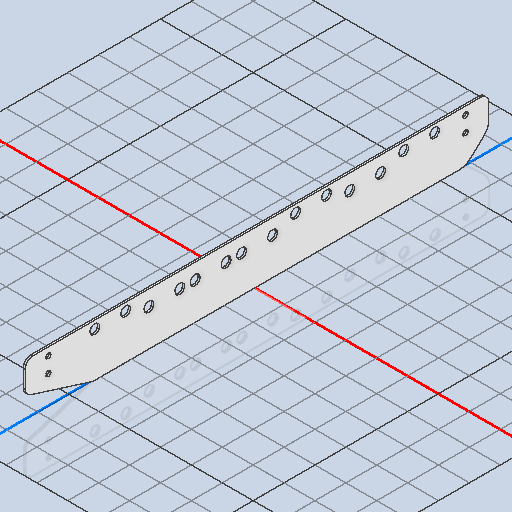
# Autodesk Inventor part: Skirt
Saved by Autodesk Inventor 2026 (Build 300175000, 175)
## iProperties
Created: 2025-04-07
Part Number: Skirt
Material: Acetal Resin, White
Document SubType Name: Modeling
Designer: avere
Density: 1.425 g/cm^3
Appearance: Smooth - White
Author: avere
Autodesk Inventor part; units mm, degrees
ref_plane "YZ Plane" through (0, 0, 0) normal (1, 0, 0) x (0, 1, 0)
ref_plane "XZ Plane" through (0, 0, 0) normal (0, 1, 0) x (-1, 0, 0)
ref_plane "XY Plane" through (0, 0, 0) normal (0, 0, 1) x (1, 0, 0)
sketch "Sketch1" plane through (0, 0, 0) normal (1, 0, 0) x (0, 1, 0)
  circle A0 centre (3.7668, 169.9011) radius 2.1844
  circle A1 centre (16.4668, 169.9011) radius 2.1844
  circle A2 centre (3.7668, -172.9989) radius 2.1844
  circle A3 centre (16.4668, -172.9989) radius 2.1844
  line L0 (16.4668, 188.9511) -> (2.0773, 188.9511)
  line L1 (-3.9805, 184.505) -> (-19.4614, 135.2476)
  line L2 (-20.0457, 131.4398) -> (-20.0457, -168.0589)
  line L3 (-16.7075, -176.6406) -> (-6.3583, -187.9307)
  line L4 (3.0036, -192.0489) -> (16.4668, -192.0489)
  line L5 (22.8168, -185.6989) -> (22.8168, 182.6011)
  arc A4 (-19.4614, 135.2476) -> (-20.0457, 131.4398) centre (-7.3457, 131.4398) ccw
  arc A5 (-20.0457, -168.0589) -> (-16.7075, -176.6406) centre (-7.3457, -168.0589) ccw
  arc A6 (-6.3583, -187.9307) -> (3.0036, -192.0489) centre (3.0036, -179.3489) ccw
  arc A7 (2.0773, 188.9511) -> (-3.9805, 184.505) centre (2.0773, 182.6011) ccw
  arc A8 (22.8168, 182.6011) -> (16.4668, 188.9511) centre (16.4668, 182.6011) ccw
  arc A9 (16.4668, -192.0489) -> (22.8168, -185.6989) centre (16.4668, -185.6989) ccw
  circle A10 centre (16.4668, 131.8011) radius 4.0005
  circle A11 centre (16.4668, 106.4011) radius 4.0005
  circle A12 centre (16.4668, -58.6989) radius 4.0005
  circle A13 centre (16.4668, -33.2989) radius 4.0005
  circle A14 centre (16.4668, -147.5989) radius 4.0005
  circle A15 centre (16.4668, -122.1989) radius 4.0005
  circle A16 centre (10.1168, 87.3511) radius 4.064
  circle A17 centre (10.1168, 61.9511) radius 4.064
  circle A18 centre (10.1168, 23.8511) radius 4.064
  circle A19 centre (10.1168, 49.2511) radius 4.064
  circle A20 centre (10.1168, -14.2489) radius 4.064
  circle A21 centre (10.1168, 11.1511) radius 4.064
  circle A22 centre (10.1168, -77.7489) radius 4.064
  circle A23 centre (10.1168, -103.1489) radius 4.064
  point P0 (0, 0)
  dimension "d16" = 12.7
  dimension "d17" = 6.35
  dimension "d18" = 6.35
  dimension "d19" = 8.001
  dimension "d20" = 25.4
  dimension "d21" = 165.1
  dimension "d22" = 254
  dimension "d23" = 8.128
  dimension "d24" = 25.4
  dimension "d25" = 38.1
  dimension "d26" = 25.4
  constraints: 24 centre point, 12 end point, 12 point on circle, 12 tangent, 5 vertical, 3 equal radius, 2 perpendicular, 1 horizontal, 14 other
  measures "d16" radius of A4
  measures "d17" radius of A7
  measures "d18" radius of A9
  measures "d19" diameter of A10
  measures "d20" distance of A10.centre A11.centre
  measures "d21" distance of A11.centre A12.centre
  measures "d22" distance of A11.centre A14.centre
  measures "d23" diameter of A16
  measures "d24" distance of A16.centre A17.centre
  measures "d25" distance of A17.centre A18.centre
  measures "d26" distance of A22.centre A23.centre
extrude "Extrusion1" add sketch "Sketch1" along normal blind 1.5875
body "Solid1"
